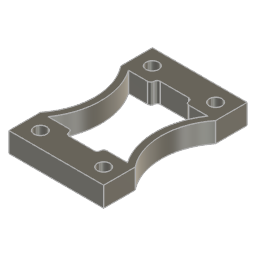
Flexure Mount (Autodesk Fusion 360 design; units mm, degrees)
part number: 2026-04-23-12-48-19-527
Autodesk Fusion 360 part; units mm, degrees
sketch "Sketch1" plane through (0, 0, 0) normal (0, 0, 1) x (1, 0, 0)
  line L0 (-7.5, 6.35) -> (7.5, 6.35)
  line L1 (7.5, 6.35) -> (7.5, 11.35)
  line L2 (7.5, 11.35) -> (-7.5, 11.35)
  line L3 (-7.5, 11.35) -> (-7.5, 6.35)
  line L4 (-7.5, 6.35) -> (7.5, 11.35) construction
  line L5 (7.5, 6.35) -> (-7.5, 11.35) construction
  line L6 (-7.5, -6.35) -> (7.5, -6.35)
  line L7 (7.5, -6.35) -> (7.5, -11.35)
  line L8 (7.5, -11.35) -> (-7.5, -11.35)
  line L9 (-7.5, -11.35) -> (-7.5, -6.35)
  line L10 (-7.5, -6.35) -> (7.5, -11.35) construction
  line L11 (7.5, -6.35) -> (-7.5, -11.35) construction
  arc A0 (-7.5, -6.35) -> (-7.5, 6.35) centre (-15.5, 0) ccw
  arc A1 (-6.2573, -6.35) -> (-6.2573, 6.35) centre (-15.5, 0) ccw
  arc A2 (7.5, 6.35) -> (7.5, -6.35) centre (15.5, 0) ccw
  arc A3 (6.2573, 6.35) -> (6.2573, -6.35) centre (15.5, 0) ccw
  circle A4 centre (-5, -8.85) radius 1
  circle A5 centre (5, -8.85) radius 1
  line L12 (-2.75, 6.35) -> (2.75, 6.35)
  line L13 (2.75, 6.35) -> (2.75, 7.35)
  line L14 (2.75, 7.35) -> (-2.75, 7.35)
  line L15 (-2.75, 7.35) -> (-2.75, 6.35)
  line L16 (-2.75, 6.35) -> (2.75, 7.35) construction
  line L17 (2.75, 6.35) -> (-2.75, 7.35) construction
  line L18 (-2.5, -6.35) -> (2.5, -6.35)
  line L19 (2.5, -6.35) -> (2.5, -7.35)
  line L20 (2.5, -7.35) -> (-2.5, -7.35)
  line L21 (-2.5, -7.35) -> (-2.5, -6.35)
  line L22 (-2.5, -6.35) -> (2.5, -7.35) construction
  line L23 (2.5, -6.35) -> (-2.5, -7.35) construction
  line L24 (0, 0) -> (-9.3045, 0) construction
  circle A6 centre (-5, 8.85) radius 1
  circle A7 centre (5, 8.85) radius 1
  point P0 (0, 8.85)
  point P1 (0, -8.85)
  point P2 (0, 6.85)
  point P3 (0, -6.85)
  dimension "d3" = 15
  dimension "d4" = 5
  dimension "d5" = 6.35
  dimension "d6" = 6.35
  dimension "d8" = 1
  dimension "d13" = 1
  dimension "d14" = 8
  dimension "d15" = 8
  dimension "d16" = 2
  dimension "d17" = 5
  dimension "d18" = 5
  dimension "d19" = 5.5
  dimension "d20" = 1
  dimension "d21" = 1
  dimension "d22" = 5
  constraint horizontal L0
  constraint perpendicular L0 L1
  constraint parallel L0 L2
  constraint parallel L1 L3
  constraint coincident L4 P0
  constraint coincident L5 P0
  constraint horizontal L6
  constraint perpendicular L6 L7
  constraint parallel L6 L8
  constraint parallel L7 L9
  constraint coincident L10 P1
  constraint coincident L11 P1
  constraint equal L0 L6
  constraint equal L3 L9
  constraint vertical L24.start P0
  constraint vertical L24.start P1
  constraint coincident L6 A1.start
  constraint coincident A0.centre A1.centre
  constraint coincident L6 A3.end
  constraint coincident L0 A3.start
  constraint coincident A2.centre A3.centre
  constraint horizontal L24.start A2.centre
  constraint coincident L6.end L7.start
  constraint coincident L0 A1.end
  constraint equal A4 A5
  constraint horizontal P1 A4.centre
  constraint horizontal P1 A5.centre
  constraint horizontal L12
  constraint perpendicular L12 L13
  constraint parallel L12 L14
  constraint parallel L13 L15
  constraint coincident L16 P2
  constraint coincident L17 P2
  constraint coincident L0 L12.start
  constraint horizontal L18
  constraint perpendicular L18 L19
  constraint parallel L18 L20
  constraint parallel L19 L21
  constraint coincident L22 P3
  constraint coincident L23 P3
  constraint coincident L6 L18.start
  constraint vertical L24.start P2
  constraint vertical L24.start P3
  constraint coincident L24.start origin
  constraint horizontal L24
  constraint symmetric A4 L24 A6
  constraint symmetric A5 L24 A7
  measures "d3" distance of L1.end L2.end
  measures "d4" distance of L0.start L2.end
  measures "d5" distance of L24.start L6
  measures "d6" distance of L24.start L0
  measures "d8" distance of A2 A3
  measures "d13" distance of A0 A1
  measures "d14" horizontal distance of L0.start A0.centre
  measures "d15" horizontal distance of L0.end A2.centre
  measures "d16" diameter of A5
  measures "d17" distance of P1 A4.centre
  measures "d18" distance of P1 A5.centre
  measures "d19" distance of L13.end L14.end
  measures "d20" distance of L12.end L13.end
  measures "d21" distance of L18.end L19.end
  measures "d22" distance of L19.end L20.end
extrude "Extrude1" add sketch "Sketch1" along normal blind 3.175 contours L0 L1 L2 L3 L13 L14 L15 | L0 L6 A0 A1 | L6 L7 L8 L9 L19 L20 L21 | L0 L6 A2 A3
fillet "Fillet1" radius 0.5 8 edges at (-2.5, -7.35, 1.5875) (-2.5, -6.35, 1.5875) (-2.75, 6.35, 1.5875) (-2.75, 7.35, 1.5875) (2.75, 6.35, 1.5875) (2.75, 7.35, 1.5875) (2.5, -6.35, 1.5875) (2.5, -7.35, 1.5875)
sketch "Sketch3" plane through (0, 0, 3.175) normal (0, 0, 1) x (-1, 0, 0)
  circle A0 centre (-5, -8.85) radius 1
  circle A1 centre (5, -8.85) radius 1
  circle A2 centre (5, 8.85) radius 1
  arc A3 (-3, 6.35) -> (-2.5, 6.85) centre (-3, 6.85) ccw
  arc A4 (-2, 7.35) -> (-2.5, 6.85) centre (-2, 6.85) ccw
  line L0 (-2, 7.35) -> (2, 7.35)
  arc A5 (2.5, 6.85) -> (2, 7.35) centre (2, 6.85) ccw
  arc A6 (2.5, 6.85) -> (3, 6.35) centre (3, 6.85) ccw
  line L1 (3, 6.35) -> (6.2573, 6.35)
  arc A7 (6.2573, 6.35) -> (6.2573, -6.35) centre (15.5, 0) ccw
  line L2 (6.2573, -6.35) -> (3.25, -6.35)
  arc A8 (3.25, -6.35) -> (2.75, -6.85) centre (3.25, -6.85) ccw
  arc A9 (2.25, -7.35) -> (2.75, -6.85) centre (2.25, -6.85) ccw
  line L3 (2.25, -7.35) -> (-2.25, -7.35)
  arc A10 (-2.75, -6.85) -> (-2.25, -7.35) centre (-2.25, -6.85) ccw
  arc A11 (-2.75, -6.85) -> (-3.25, -6.35) centre (-3.25, -6.85) ccw
  line L4 (-3.25, -6.35) -> (-6.2573, -6.35)
  arc A12 (-6.2573, -6.35) -> (-6.2573, 6.35) centre (-15.5, 0) ccw
  line L5 (-6.2573, 6.35) -> (-3, 6.35)
  circle A13 centre (-5, 8.85) radius 1
  line L6 (-7.5, -11.35) -> (7.5, -11.35)
  line L7 (7.5, -11.35) -> (7.5, -6.35)
  arc A14 (7.5, 6.35) -> (7.5, -6.35) centre (15.5, 0) ccw
  line L8 (7.5, 6.35) -> (7.5, 11.35)
  line L9 (7.5, 11.35) -> (-7.5, 11.35)
  line L10 (-7.5, 11.35) -> (-7.5, 6.35)
  arc A15 (-7.5, -6.35) -> (-7.5, 6.35) centre (-15.5, 0) ccw
  line L11 (-7.5, -6.35) -> (-7.5, -11.35)
  circle A16 centre (5, 8.85) radius 1
  constraint concentric A2 A16
equation "d6 = d5"
equation "d8 = d13"
equation "d11 = 0'- 1/8\""
equation "d15 = d14"
equation "d18 = d17"
equation "d21 = d20"
